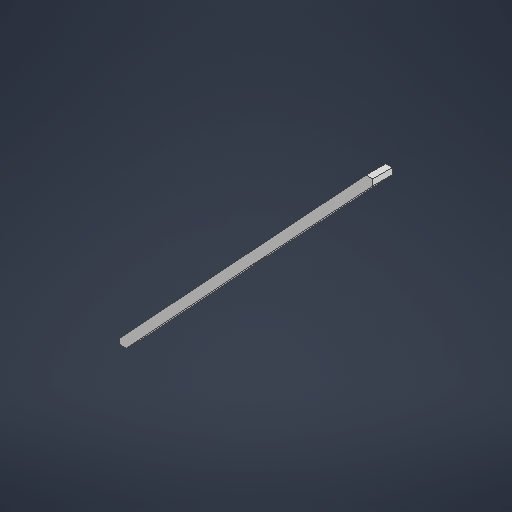
# Autodesk Inventor part: S_2x4x65.795
Saved by Autodesk Inventor 2026 (Build 300175000, 175)
## iProperties
Created: 2025-09-02
Part Number: S_2x4x65.795
Material: Generic
Document SubType Name: Modeling
Designer: trott
Density: 1 g/cm^3
Appearance: Default
Author: trott
Autodesk Inventor part; units mm, degrees
ref_plane "YZ Plane" through (0, 0, 0) normal (1, 0, 0) x (0, 1, 0)
ref_plane "XZ Plane" through (0, 0, 0) normal (0, 1, 0) x (-1, 0, 0)
ref_plane "XY Plane" through (0, 0, 0) normal (0, 0, 1) x (1, 0, 0)
sketch "Sketch1" plane through (0, 0, 0) normal (0, 0, 1) x (1, 0, 0)
  line L0 (-571.5, -609.6) -> (571.5, -609.6)
  line L1 (571.5, -609.6) -> (571.5, 609.6)
  line L2 (571.5, 609.6) -> (-571.5, 609.6)
  line L3 (-571.5, 609.6) -> (-571.5, -609.6)
  line L4 (-571.5, -609.6) -> (571.5, 609.6) construction
  line L5 (571.5, -609.6) -> (-571.5, 609.6) construction
  line L6 (13.0291, -13.8977) -> (-13.0291, 13.8977)
  line L7 (13.0291, -13.8977) -> (571.5, 581.8046)
  line L8 (-13.0291, 13.8977) -> (541.8516, 609.6)
  line L9 (13.0291, -13.8977) -> (-541.8516, -609.6)
  line L10 (-13.0291, 13.8977) -> (-571.5, -585.659)
  point P0 (0, 0)
  dimension "d3" = 38.1
  constraints: 22 end point, 6 point on line, 4 parallel, 3 midpoint, 1 horizontal, 1 perpendicular
  measures "d3" distance of L6.start L6.end
extrude "Extrusion1" add sketch "Sketch1" along normal blind 88.9 contours L3 L10 L6 L9 L0 | L6 L8 L2 L1 L7
body "Solid1"
